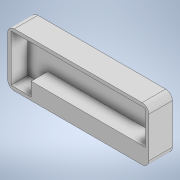
# Autodesk Inventor part: Maccaron_Filter
Saved by Autodesk Inventor 2021 (Build 250183000, 183)
## iProperties
Created: 2024-05-18
Part Number: Maccaron_Filter
Material: Generic
Document SubType Name: Modeling
Designer: Lukas
Density: 1 g/cm^3
Appearance: Default
Author: Lukas
Autodesk Inventor part; units mm, degrees
ref_plane "YZ Plane" through (0, 0, 0) normal (1, 0, 0) x (0, 1, 0)
ref_plane "XZ Plane" through (0, 0, 0) normal (0, 1, 0) x (-1, 0, 0)
ref_plane "XY Plane" through (0, 0, 0) normal (0, 0, 1) x (1, 0, 0)
sketch "Sketch1" plane through (0, 0, 0) normal (0, 0, 1) x (1, 0, 0)
  line L0 (-21, 8) -> (21, 8)
  line L1 (21, 8) -> (21, -8)
  line L2 (21, -8) -> (-21, -8)
  line L3 (-21, -8) -> (-21, 8)
  point P0 (0, 0)
  point P1 (0, 8)
  point P2 (-21, 0)
  dimension "d11" = 42
  dimension "d12" = 16
  constraints: 8 end point, 2 midpoint, 2 parallel, 1 horizontal, 1 horizontal alignment, 1 perpendicular, 1 vertical alignment
  measures "d11" distance of L0.start L0.end
  measures "d12" distance of L0.end L1.end
extrude "Extrusion1" add sketch "Sketch1" along normal blind 2
sketch "Sketch2" plane through (0, 0, 2) normal (0, 0, 1) x (1, 0, 0)
  line L0 (-21, -8) -> (21, -8) projected
  line L1 (21, -8) -> (21, 8) projected
  line L2 (21, 8) -> (-21, 8) projected
  line L3 (-21, 8) -> (-21, -8) projected
  line L4 (-20, 7) -> (20, 7)
  line L5 (20, 7) -> (20, -3)
  line L6 (20, -3) -> (-14, -3)
  line L7 (-14, -3) -> (-14, -7)
  line L8 (-14, -7) -> (-20, -7)
  line L9 (-20, -7) -> (-20, 7)
  point P0 (0, 0)
  point P1 (-20, 0)
  point P2 (0, 7)
  dimension "d13" = 40
  dimension "d14" = 10
  dimension "d15" = 6
  dimension "d16" = 4
  constraints: 12 end point, 5 perpendicular, 2 midpoint, 1 horizontal, 1 horizontal alignment, 1 vertical alignment
  measures "d13" distance of L4.start L4.end
  measures "d14" distance of L4.end L5.end
  measures "d15" distance of L7.end L8.end
  measures "d16" distance of L6.end L7.end
extrude "Extrusion3" add sketch "Sketch2" along normal blind 5
fillet "Fillet2" radius 2 4 edges at (-21, 8, 3.5) (-21, -8, 3.5) (21, -8, 3.5) (21, 8, 3.5)
body "Solid1"
